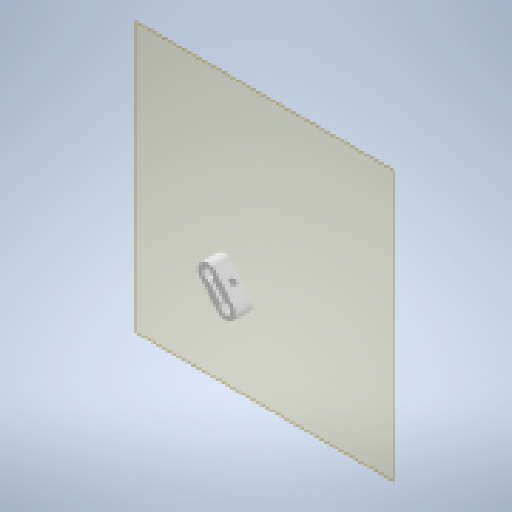
# Autodesk Inventor part: rail_holder
Saved by Autodesk Inventor 2024 (Build 280153000, 153)
## iProperties
Created: 2026-02-14
Part Number: rail_holder
Material: Generic
Document SubType Name: Modeling
Designer: SEMEN
Density: 1 g/cm^3
Appearance: Default
Author: SEMEN
Autodesk Inventor part; units mm, degrees
ref_plane "YZ Plane" through (0, 0, 0) normal (1, 0, 0) x (0, 1, 0)
ref_plane "XZ Plane" through (0, 0, 0) normal (0, 1, 0) x (-1, 0, 0)
ref_plane "XY Plane" through (0, 0, 0) normal (0, 0, 1) x (1, 0, 0)
ref_plane "Work Plane1" through (60.6116, 29.9097, 55) normal (0, 0, 1) x (1, 0, 0)
sketch "Sketch1" plane through (60.6116, 29.9097, 55) normal (0, 0, 1) x (1, 0, 0)
  circle A0 centre (-11.75, -9.4206) radius 1.5 projected
  circle A1 centre (-6.6055, -15.5471) radius 1.5 projected
  arc A2 (-9.4525, -7.4914) -> (-14.0475, -11.3498) centre (-11.75, -9.4206) ccw
  arc A3 (-8.903, -17.4763) -> (-4.3081, -13.618) centre (-6.6055, -15.5471) ccw
  line L0 (-9.4525, -7.4914) -> (-4.3081, -13.618)
  line L1 (-8.903, -17.4763) -> (-14.0475, -11.3498)
  line L2 (-11.489, -10.8977) -> (-8.0153, -15.0346)
  line L3 (-10.3403, -9.9331) -> (-6.8665, -14.07)
  line L4 (-11.75, -9.4206) -> (-6.6055, -15.5471) construction
  point P0 (-60.6116, -29.9097)
  dimension "d0" = 6
  dimension "d1" = 6
  dimension "d2" = 1.5
  constraints: 10 end point, 8 point on circle, 4 tangent, 2 centre point, 2 coincident, 1 parallel, 1 other
  measures "d0" diameter of A2
  measures "d1" diameter of A3
  measures "d2" distance between parallel lines of L3 L2
extrude "Extrusion1" add sketch "Sketch1" along normal blind 4
sketch "Sketch2" plane through (51.7087, 12.4334, 55) normal (-0.7658175, -0.643058, 0) x (0, 0, 1)
  line L0 (4, 0) -> (4, 8) projected
  line L1 (4, 4) -> (0, 4) construction
  line L2 (0, 6.701) -> (0, 1.299) projected
  line L3 (0, 0) -> (4, 0) projected
  line L4 (2, 0) -> (2, 8) construction
  line L5 (0, 8) -> (4, 8) projected
  point P0 (-55, 23.7299)
  point P1 (2, 4)
  constraints: 5 midpoint, 4 end point
hole "Hole1" at (49.1364, 15.4967, 57) direction (0.7658175, 0.643058, 0) diameter 2.4 end through all clearance for "Countersunk Head GOST 12876-67" size "M2" standard "GOST"
body "Solid1"
